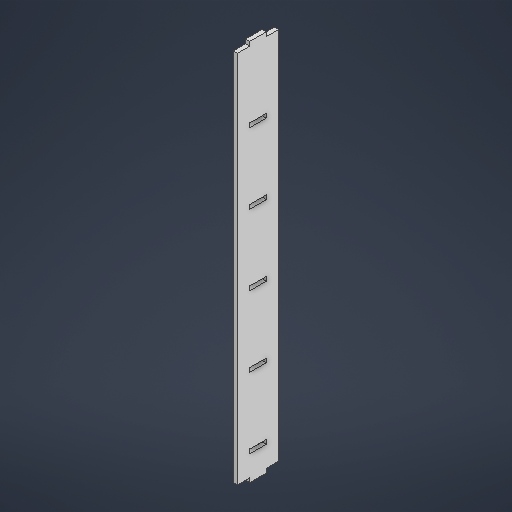
# Autodesk Inventor part: Part2
Saved by Autodesk Inventor 2026 (Build 300175050, 175E)
## iProperties
Created: 2025-06-06
Part Number: Part2
Material: Generic
Document SubType Name: Modeling
Designer: HP
Density: 1 g/cm^3
Appearance: Default
Author: HP
Autodesk Inventor part; units mm, degrees
ref_plane "YZ Plane" through (0, 0, 0) normal (1, 0, 0) x (0, 1, 0)
ref_plane "XZ Plane" through (0, 0, 0) normal (0, 1, 0) x (-1, 0, 0)
ref_plane "XY Plane" through (0, 0, 0) normal (0, 0, 1) x (1, 0, 0)
sketch "Sketch1" plane through (0, 0, 0) normal (1, 0, 0) x (0, 1, 0)
  line L0 (0, 0) -> (450, 0)
  line L1 (450, 0) -> (450, -50)
  line L2 (450, -50) -> (0, -50)
  line L3 (0, -50) -> (0, 0)
  dimension "d0" = 450
  dimension "d1" = 50
  constraints: 8 end point, 2 parallel, 1 horizontal, 1 perpendicular
  measures "d0" distance of L1.end L2.end
  measures "d1" distance of L0.end L1.end
extrude "Extrusion1" add sketch "Sketch1" along normal blind 5
sketch "Sketch2" plane through (0, 450, 0) normal (0, 1, 0) x (1, 0, 0)
  line L0 (0, 50) -> (0, 0) projected
  line L1 (0, 35) -> (5, 35)
  line L2 (5, 35) -> (5, 15)
  line L3 (5, 15) -> (0, 15)
  line L4 (0, 15) -> (0, 35)
  line L5 (0, 50) -> (5, 50) projected
  point P0 (2.5, 15)
  point P1 (2.5, 35)
  point P2 (2.5, 50)
  point P3 (0, 15)
  dimension "d4" = 5
  dimension "d5" = 20
  dimension "d6" = 15
  constraints: 8 end point, 3 midpoint, 2 parallel, 1 horizontal, 1 perpendicular, 1 point on line
  measures "d4" distance of L2.end L3.end
  measures "d5" distance of point (2.5, 15) point (2.5, 35)
  measures "d6" distance of point (2.5, 50) point (2.5, 35)
extrude "Extrusion2" add sketch "Sketch2" along normal blind 5
sketch "Sketch3" plane through (0, 0, -50) normal (0, -1, 0) x (1, 0, 0)
  line L0 (5, 50) -> (5, 0) projected
  line L1 (0, 50) -> (0, 0) projected
  line L2 (5, 35) -> (0, 35)
  line L3 (0, 35) -> (0, 15)
  line L4 (0, 15) -> (5, 15)
  line L5 (5, 15) -> (5, 35)
  line L6 (0, 50) -> (5, 50) projected
  point P0 (2.5, 50)
  point P1 (2.5, 35)
  point P2 (0, 35)
  dimension "d9" = 20
  dimension "d10" = 15
  constraints: 8 end point, 2 midpoint, 2 parallel, 2 point on line, 1 horizontal, 1 perpendicular
  measures "d9" distance of L3.end L2.end
  measures "d10" distance of point (2.5, 50) point (2.5, 35)
extrude "Extrusion3" add sketch "Sketch3" along normal blind 5 contours L0 L4 L1 L2
sketch "Sketch4" plane through (5, 0, 0) normal (1, 0, 0) x (0, 0, -1)
  line L0 (15, 370) -> (35, 370)
  line L1 (35, 370) -> (35, 365)
  line L2 (35, 365) -> (15, 365)
  line L3 (15, 365) -> (15, 370)
  line L4 (15, 450) -> (0, 450) projected
  line L5 (0, 450) -> (0, 0) projected
  line L6 (15, 285) -> (35, 285)
  line L7 (35, 285) -> (35, 280)
  line L8 (35, 280) -> (15, 280)
  line L9 (15, 280) -> (15, 285)
  line L10 (50, 0) -> (50, 450) projected
  line L11 (15, 200) -> (35, 200)
  line L12 (35, 200) -> (35, 195)
  line L13 (35, 195) -> (15, 195)
  line L14 (15, 195) -> (15, 200)
  line L15 (15, 115) -> (35, 115)
  line L16 (35, 115) -> (35, 110)
  line L17 (35, 110) -> (15, 110)
  line L18 (15, 110) -> (15, 115)
  line L19 (15, 30) -> (35, 30)
  line L20 (35, 30) -> (35, 25)
  line L21 (35, 25) -> (15, 25)
  line L22 (15, 25) -> (15, 30)
  point P0 (7.5, 450)
  point P1 (25, 370)
  point P2 (15, 367.5)
  point P3 (15, 282.5)
  point P4 (35, 282.5)
  point P5 (25, 365)
  point P6 (25, 285)
  point P7 (15, 197.5)
  point P8 (35, 197.5)
  point P9 (15, 112.5)
  point P10 (35, 112.5)
  point P11 (25, 195)
  point P12 (25, 115)
  point P13 (25, 110)
  point P14 (25, 30)
  point P15 (15, 27.5)
  point P16 (35, 27.5)
  dimension "d13" = 20
  dimension "d14" = 5
  dimension "d15" = 80
  dimension "d16" = 15
  dimension "d17" = 5
  dimension "d18" = 15
  dimension "d19" = 15
  dimension "d20" = 80
  dimension "d21" = 5
  dimension "d22" = 80
  dimension "d23" = 5
  dimension "d24" = 15
  dimension "d25" = 15
  dimension "d26" = 80
  dimension "d27" = 5
  dimension "d28" = 80
  dimension "d29" = 15
  dimension "d30" = 15
  constraints: 40 end point, 17 midpoint, 10 parallel, 5 horizontal, 5 perpendicular, 2 vertical alignment
  measures "d13" distance of L1.end L2.end
  measures "d14" distance of L0.end L1.end
  measures "d15" vertical distance of point (7.5, 450) point (25, 370)
  measures "d16" distance from line of L5 point (15, 367.5)
  measures "d17" distance of L6.end L7.end
  measures "d18" distance from line of L5 point (15, 282.5)
  measures "d19" distance from line of L10 point (35, 282.5)
  measures "d20" distance of point (25, 365) point (25, 285)
  measures "d21" distance of L11.end L12.end
  measures "d22" distance between parallel lines of L11 L8
  measures "d23" distance of L15.end L16.end
  measures "d24" distance from line of L5 point (15, 112.5)
  measures "d25" distance from line of L10 point (35, 112.5)
  measures "d26" distance of point (25, 195) point (25, 115)
  measures "d27" distance of L19.end L20.end
  measures "d28" distance of point (25, 110) point (25, 30)
  measures "d29" distance from line of L5 point (15, 27.5)
  measures "d30" distance from line of L10 point (35, 27.5)
extrude "Extrusion4" cut sketch "Sketch4" against normal blind 5
body "Solid1"
